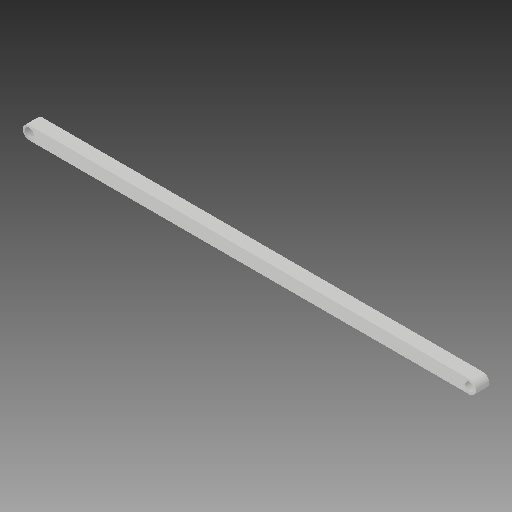
# Autodesk Inventor part: L4
Saved by Autodesk Inventor 2019 (Build 230136000, 136)
## iProperties
Created: 2020-03-18
Part Number: L4
Material: Generic
Document SubType Name: Modeling
Designer: Pulag
Density: 1 g/cm^3
Appearance: Default
Author: Pulag
Autodesk Inventor part; units mm, degrees
ref_plane "YZ Plane" through (0, 0, 0) normal (1, 0, 0) x (0, 1, 0)
ref_plane "XZ Plane" through (0, 0, 0) normal (0, 1, 0) x (-1, 0, 0)
ref_plane "XY Plane" through (0, 0, 0) normal (0, 0, 1) x (1, 0, 0)
sketch "Sketch1" plane through (0, 0, 0) normal (0, 0, 1) x (1, 0, 0)
  line L0 (0, 0) -> (100, 0)
  line L1 (100, 3) -> (0, 3)
  arc A0 (0, 3) -> (0, 0) centre (0, 1.5) ccw
  arc A1 (100, 0) -> (100, 3) centre (100, 1.5) ccw
  circle A2 centre (0, 1.5) radius 1
  circle A3 centre (100, 1.5) radius 1
  dimension "d0" = 2
  dimension "d1" = 2
  dimension "d2" = 100
  constraints: 4 centre point, 4 end point, 4 point on circle, 4 tangent, 2 coincident, 1 horizontal, 1 parallel
  measures "d0" diameter of A2
  measures "d1" diameter of A3
  measures "d2" distance of A1.centre A0.centre
extrude "Extrusion1" add sketch "Sketch1" along normal blind 3
body "Solid1"
